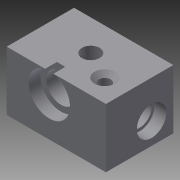
# Autodesk Inventor part: FxDrill_02
Saved by Autodesk Inventor 2015 SP2 (Build 190223200, 223)
## iProperties
Created: 2017-09-03
Part Number: FxDrill_02
Material: Generisch
Document SubType Name: Modeling
Designer: jensp
Density: 1 g/cm^3
Appearance: Vorgabe
Author: jensp
Autodesk Inventor part; units mm, degrees
ref_plane "YZ Plane" through (0, 0, 0) normal (1, 0, 0) x (0, 1, 0)
ref_plane "XZ Plane" through (0, 0, 0) normal (0, 1, 0) x (-1, 0, 0)
ref_plane "XY Plane" through (0, 0, 0) normal (0, 0, 1) x (1, 0, 0)
sketch "Skizze1" plane through (0, 0, 0) normal (0, 0, 1) x (1, 0, 0)
  line L0 (-8.0351, 5.2058) -> (8.7518, 5.2058)
  line L1 (8.7518, 5.2058) -> (8.7518, -6.1866)
  line L2 (8.7518, -6.1866) -> (-8.0351, -6.1866)
  line L3 (-8.0351, -6.1866) -> (-8.0351, 5.2058)
  point P0 (0, 0)
  constraints: 8 end point, 2 parallel, 1 horizontal, 1 perpendicular
extrude "Extrusion1" add sketch "Skizze1" along normal blind 10
sketch "Skizze2" plane through (0, 0, 10) normal (0, 0, 1) x (1, 0, 0)
  point P0 (0, 0)
hole "Drill01" at (0, 0, 10) direction (0, 0, -1) diameter 3 depth 8 tip angle 120
hole "Drill02" at (8.7518, 1.5333, 3.6521) direction (-1, 0, 0) diameter 4 depth 4 tip angle 118 counterbore diameter 5 counterbore depth 2
hole "Drill03" at (-0.835, -6.1866, 6.5728) direction (0, 1, 0) diameter 5 depth 6 tip angle 118 counterbore diameter 7 counterbore depth 2
hole "Drill04" at (4.8061, -2.4326, 10) direction (0, 0, -1) diameter 2 depth 6 tip angle 118 countersink diameter 3.5 countersink angle 90
